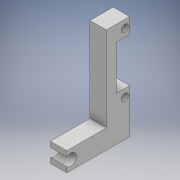
# Autodesk Inventor part: Laser_Holder_1
Saved by Autodesk Inventor 2017 (Build 210142000, 142)
## iProperties
Created: 2017-05-03
Part Number: Laser_Holder_1
Material: Generic
Document SubType Name: Modeling
Designer: willt
Density: 1 g/cm^3
Appearance: Default
Author: willt
Autodesk Inventor part; units mm, degrees
ref_plane "YZ Plane" through (0, 0, 0) normal (1, 0, 0) x (0, 1, 0)
ref_plane "XZ Plane" through (0, 0, 0) normal (0, 1, 0) x (-1, 0, 0)
ref_plane "XY Plane" through (0, 0, 0) normal (0, 0, 1) x (1, 0, 0)
sketch "Sketch1" plane through (0, 0, 0) normal (1, 0, 0) x (0, 1, 0)
  line L0 (0, 0) -> (0, -8)
  line L1 (0, -8) -> (-7, -8)
  line L2 (-7, -8) -> (-7, -31)
  line L3 (-7, -31) -> (0, -31)
  line L4 (-12, 0) -> (0, 0)
  line L5 (0, -4) -> (-2.5, -4) construction
  circle A0 centre (-2.5, -4) radius 1.875
  line L6 (0, -31) -> (-2.5, -31) construction
  line L7 (-2.5, -31) -> (-2.5, -35) construction
  circle A1 centre (-2.5, -35) radius 1.875
  line L8 (-30.5, -54) -> (0, -54)
  arc A2 (-32.5, -51.1957) -> (-32.5, -46.8043) centre (-30.5, -49) ccw
  line L9 (-30.5, -44) -> (-32.5, -44)
  line L10 (-32.5, -44) -> (-32.5, -46.8043)
  line L11 (-30.5, -54) -> (-32.5, -54)
  line L12 (-32.5, -54) -> (-32.5, -51.1957)
  line L13 (-12, -44) -> (-30.5, -44)
  line L14 (0, -31) -> (0, -54)
  line L15 (-12, 0) -> (-12, -44)
  dimension "d0" = 8
  dimension "d1" = 7
  dimension "d2" = 23
  dimension "d5" = 2.5
  dimension "d6" = 3.75
  dimension "d7" = 4
  dimension "d8" = 3.75
  dimension "d10" = 30.5
  dimension "d11" = 10
  dimension "d13" = 2
  constraints: 32 end point, 6 perpendicular, 4 point on line, 3 centre point, 3 coincident, 3 horizontal, 2 parallel, 2 point on circle, 2 vertical, 1 midpoint
  measures "d0" distance of L0.start L0.end
  measures "d1" distance of L0.end L1.end
  measures "d2" distance of L1.end L2.end
  measures "d5" distance of L5.start L5.end
  measures "d6" diameter of A0
  measures "d7" distance of L6.end L7.end
  measures "d8" diameter of A1
  measures "d10" distance of L8.end L8.start
  measures "d11" distance of L8.start L9.start
  measures "d13" distance of L9.start L9.end
extrude "Extrusion1" add sketch "Sketch1" along normal blind 8.5
body "Solid1"
